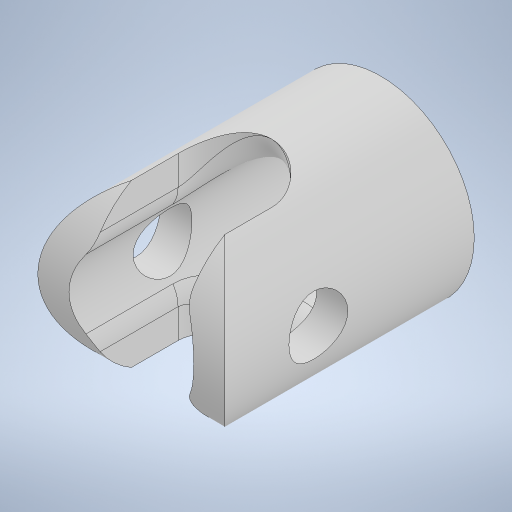
# Autodesk Inventor part: Anchor
Saved by Autodesk Inventor 2023.2 (Build 272271000, 271)
## iProperties
Created: 2024-02-03
Part Number: Anchor
Material: Generic
Document SubType Name: Modeling
Designer: Nathan Cai
Density: 1 g/cm^3
Appearance: Default
Author: Nathan Cai
Autodesk Inventor part; units mm, degrees
ref_plane "YZ Plane" through (0, 0, 0) normal (1, 0, 0) x (0, 1, 0)
ref_plane "XZ Plane" through (0, 0, 0) normal (0, 1, 0) x (-1, 0, 0)
ref_plane "XY Plane" through (0, 0, 0) normal (0, 0, 1) x (1, 0, 0)
sketch "Sketch1" plane through (0, 0, 0) normal (0, 0, 1) x (1, 0, 0)
  circle A0 centre (0, 0) radius 3.175
  circle A1 centre (0, 0) radius 4.7625
  dimension "d0" = 6.35
  dimension "d1" = 9.525
  constraints: 2 centre point, 2 coincident
  measures "d0" diameter of A0
  measures "d1" diameter of A1
extrude "Extrusion1" add sketch "Sketch1" along normal blind 12.7
sketch "Sketch5" plane through (0, 0, 0) normal (1, 0, 0) x (0, 1, 0)
  circle A0 centre (0, 7.9375) radius 4.7625
  line L0 (4.7625, 12.7) -> (-4.7625, 12.7) projected
  line L1 (0, 12.7) -> (0, 0) construction
  circle A1 centre (0, 7.9375) radius 1.5
  line L2 (4.7625, 12.7) -> (-4.7625, 12.7) projected
  line L3 (4.7625, 0) -> (-4.7625, 0) projected
  line L4 (4.7625, 0) -> (4.7625, 12.7) projected
  line L5 (-4.7625, 0) -> (-4.7625, 12.7) projected
  point P0 (-4.7625, 7.9375)
  point P1 (0, 12.7)
  point P2 (4.7625, 7.9375)
  dimension "d24" = 9.525
  dimension "d25" = 3
  constraints: 2 centre point, 2 end point, 1 coincident, 1 midpoint, 1 point on line, 1 tangent, 1 vertical
  measures "d24" diameter of A0
  measures "d25" diameter of A1
extrude "Extrusion4" cut sketch "Sketch5" along normal through all both and the other way through all contours A0 L0 L4 | A0 L5 L0 | A1
sketch "Sketch6" plane through (0, 0, 0) normal (0, 1, 0) x (-1, 0, 0)
  line L0 (-4.7625, 12.7) -> (4.7625, 12.7) construction
  line L1 (4.7625, 12.7) -> (-4.7625, 12.7)
  line L2 (0, 12.7) -> (0, 0) construction
  line L3 (0, 12.7) -> (0, 7.9375) construction
  line L4 (-2.3812, 12.7) -> (-2.3812, 7.9375)
  line L5 (2.3813, 7.9375) -> (2.3812, 12.7)
  arc A0 (2.3812, 12.7) -> (-2.3812, 12.7) centre (0, 12.7) ccw
  arc A1 (-2.3812, 7.9375) -> (2.3813, 7.9375) centre (0, 7.9375) ccw
  point P0 (0, 10.3187)
  dimension "d29" = 4.7625
  dimension "d30" = 4.7625
  constraints: 12 end point, 4 point on circle, 4 tangent, 3 point on line, 2 centre point, 2 midpoint, 1 parallel, 1 vertical
  measures "d29" distance of L2.start L3.end
  measures "d30" diameter of A1
extrude "Extrusion5" cut sketch "Sketch6" along normal through all both and the other way through all
fillet "Fillet2" radius 1.5875 2 edges at (-0.0026, -3.175, 5.5563) (0.0026, 3.175, 5.5563)
body "Solid1"
